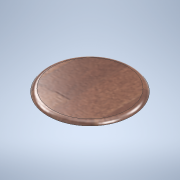
# Autodesk Inventor part: CapTop-ver1-1111-2021
Saved by Autodesk Inventor 2021 (Build 250183000, 183)
## iProperties
Created: 2021-03-03
Part Number: CapTop-ver1-1111-2021
Material: Generic
Document SubType Name: Modeling
Designer: CMurray
Density: 1 g/cm^3
Appearance: Default
Author: CMurray
Autodesk Inventor part; units mm, degrees
ref_plane "YZ Plane" through (0, 0, 0) normal (1, 0, 0) x (0, 1, 0)
ref_plane "XZ Plane" through (0, 0, 0) normal (0, 1, 0) x (-1, 0, 0)
sketch "Sketch1" plane through (0, 0, 0) normal (0, 1, 0) x (-1, 0, 0)
  circle A0 centre (0, 0) radius 107.95
  dimension "d0" = 215.9
  constraints: 1 centre point, 1 coincident
  measures "d0" diameter of A0
extrude "Extrusion1" add sketch "Sketch1" along normal blind 7.62
ref_plane "Work Plane1" through (0, 0, 107.95) normal (0, 0, 1) x (1, 0, 0)
fillet "Fillet1" radius 12.7 1 edges at (107.95, 7.62, 0)
body "Solid1"
